Autodesk Fusion 360 part; units mm, degrees
note: some values were not read from the file. Chosen so that the rebuilt part matches the saved one: which bodies a step acts on; which face or edge a step refers to. Set by a fixed rule: which sketch regions a step uses.
(part 2 of 2)
sketch "Sketch18" plane through (0, 0, 282) normal (0, 0, 1) x (1, 0, 0)
  line L0 (0.3171, 299.31) -> (-8.3702, 323.1782)
  line L1 (-8.3702, 323.1782) -> (15.4979, 331.8655)
  line L2 (15.4979, 331.8655) -> (24.1853, 307.9973)
  line L3 (23.3949, 293.8753) -> (29.573, 307.8136)
  line L4 (29.573, 307.8136) -> (18.4863, 338.2741)
  line L5 (18.4863, 338.2741) -> (-14.7788, 326.1666)
  line L6 (-14.7788, 326.1666) -> (-3.6921, 295.7061)
  line L7 (-3.6921, 295.7061) -> (10, 289)
  line L8 (19.5766, 262.6886) -> (13.3984, 248.7503)
  line L9 (13.3984, 248.7503) -> (24.4851, 218.2899)
  line L10 (24.4851, 218.2899) -> (57.7502, 230.3974)
  line L11 (57.7502, 230.3974) -> (46.6635, 260.8578)
  line L12 (46.6635, 260.8578) -> (32.9714, 267.5639)
  line L13 (42.6543, 257.2539) -> (51.3417, 233.3857)
  line L14 (51.3417, 233.3857) -> (27.4735, 224.6984)
  line L15 (27.4735, 224.6984) -> (18.7862, 248.5666)
  line L16 (22.4806, 294.2806) -> (28.4955, 307.8504)
  line L17 (28.4955, 307.8504) -> (17.8886, 336.9924)
  line L18 (17.8886, 336.9924) -> (-13.4971, 325.5689)
  line L19 (-13.4971, 325.5689) -> (-2.8903, 296.4269)
  line L20 (-2.8903, 296.4269) -> (10.4399, 289.8981)
  line L21 (21.5664, 294.6858) -> (27.4179, 307.8871)
  line L22 (27.4179, 307.8871) -> (17.291, 335.7107)
  line L23 (17.291, 335.7107) -> (-12.2154, 324.9712)
  line L24 (-12.2154, 324.9712) -> (-2.0884, 297.1477)
  line L25 (-2.0884, 297.1477) -> (10.8797, 290.7961)
  line L26 (20.6522, 295.091) -> (26.3404, 307.9238)
  line L27 (26.3404, 307.9238) -> (16.6933, 334.4289)
  line L28 (16.6933, 334.4289) -> (-10.9337, 324.3735)
  line L29 (-10.9337, 324.3735) -> (-1.2866, 297.8685)
  line L30 (-1.2866, 297.8685) -> (11.3196, 291.6942)
  line L31 (19.738, 295.4962) -> (25.2628, 307.9606)
  line L32 (25.2628, 307.9606) -> (16.0956, 333.1472)
  line L33 (16.0956, 333.1472) -> (-9.652, 323.7759)
  line L34 (-9.652, 323.7759) -> (-0.4848, 298.5892)
  line L35 (-0.4848, 298.5892) -> (11.7594, 292.5923)
  line L36 (19.738, 295.4962) -> (23.3949, 293.8753)
  line L37 (11.7594, 292.5923) -> (10, 289)
  line L38 (21.0393, 262.0402) -> (15.1225, 248.6915)
  line L39 (15.1225, 248.6915) -> (25.4414, 220.3406)
  line L40 (25.4414, 220.3406) -> (55.6995, 231.3536)
  line L41 (55.6995, 231.3536) -> (45.3806, 259.7046)
  line L42 (45.3806, 259.7046) -> (32.2676, 266.127)
  line L43 (22.5021, 261.3919) -> (16.8466, 248.6327)
  line L44 (16.8466, 248.6327) -> (26.3977, 222.3913)
  line L45 (26.3977, 222.3913) -> (53.6487, 232.3099)
  line L46 (53.6487, 232.3099) -> (44.0977, 258.5513)
  line L47 (44.0977, 258.5513) -> (31.5639, 264.6901)
  line L48 (23.9648, 260.7435) -> (18.5706, 248.574)
  line L49 (18.5706, 248.574) -> (27.3539, 224.4421)
  line L50 (27.3539, 224.4421) -> (51.598, 233.2662)
  line L51 (51.598, 233.2662) -> (42.8147, 257.3981)
  line L52 (42.8147, 257.3981) -> (30.8601, 263.2532)
  line L53 (25.4275, 260.0952) -> (20.2947, 248.5152)
  line L54 (20.2947, 248.5152) -> (28.3102, 226.4928)
  line L55 (28.3102, 226.4928) -> (49.5473, 234.2225)
  line L56 (49.5473, 234.2225) -> (41.5318, 256.2448)
  line L57 (41.5318, 256.2448) -> (30.1563, 261.8163)
  line L58 (30.1563, 261.8163) -> (32.9714, 267.5639)
  line L59 (25.4275, 260.0952) -> (19.5766, 262.6886)
  line L60 (24.1853, 307.9973) -> (18.8238, 295.9015)
  line L61 (18.8238, 295.9015) -> (19.738, 295.4962)
  line L62 (0.3171, 299.31) -> (12.1993, 293.4903)
  line L63 (12.1993, 293.4903) -> (11.7594, 292.5923)
  line L64 (25.4275, 260.0952) -> (24.1476, 260.6625)
  line L65 (24.1476, 260.6625) -> (18.7862, 248.5666)
  line L66 (30.1563, 261.8163) -> (30.7721, 263.0736)
  line L67 (30.7721, 263.0736) -> (42.6543, 257.2539)
  dimension "d128" = 1
  dimension "d129" = 2
  dimension "d130" = 3
  dimension "d131" = 4
  dimension "d132" = 1.6
  dimension "d133" = 3.2
  dimension "d134" = 4.8
  dimension "d135" = 6.4
extrude "Extrude26" add sketch "Sketch18" against normal up to surface (127 mm away) separate body contours L3 L4 L5 L6 L7 L16 L17 L18 L19 L20 L36 L37 | L8 L9 L10 L11 L12 L38 L39 L40 L41 L42 L58 L59 makes body 48 at (7.3979, 334.2382, 239.6667) makes body 49 at (35.5735, 222.3257, 239.6667)
delete_body "RemoveBody32" bodies 23
delete_body "RemoveBody33" bodies 18
extrude "Extrude27" add sketch "Sketch18" against normal up to surface (127 mm away) separate body contours L16 L17 L18 L19 L20 L21 L22 L23 L24 L25 L36 L37 | L38 L39 L40 L41 L42 L43 L44 L45 L46 L47 L58 L59 makes body 50 at (35.5274, 224.0116, 239.6667) makes body 51 at (7.4267, 333.1845, 239.6667)
extrude "Extrude28" add sketch "Sketch18" against normal up to surface (127 mm away) separate body contours L21 L22 L23 L24 L25 L26 L27 L28 L29 L30 L36 L37 | L43 L44 L45 L46 L47 L48 L49 L50 L51 L52 L58 L59 makes body 52 at (7.4555, 332.1308, 197.3333) makes body 53 at (35.4814, 225.6975, 239.6667)
extrude "Extrude29" add sketch "Sketch18" against normal up to surface (127 mm away) separate body contours L26 L27 L28 L29 L30 L31 L32 L33 L34 L35 L36 L37 | L13 L14 L15 L48 L49 L50 L51 L52 L58 L59 L65 L67 | L13 L14 L15 L53 L54 L55 L56 L57 L58 L59 L64 L65 L66 L67 makes body 54 at (35.4353, 227.3834, 239.6667) makes body 55 at (7.4843, 331.0771, 239.6667)
extrude "Extrude30" add sketch "Sketch18" against normal up to surface (127 mm away) separate body contours L0 L1 L2 L31 L32 L33 L34 L35 L60 L61 L62 L63 | L13 L14 L15 L53 L54 L55 L56 L57 L58 L59 L64 L65 L66 L67 makes body 56 at (43.3856, 230.49, 197.3333) makes body 57 at (7.5131, 330.0234, 239.6667)
pattern_circular "C-Pattern2" count 5 over 360 about axis through (0, 205, 400) along (0, 0, -1) of bodies 49 50 53 54 56 38 makes body 58 at (60.6403, 201.5558, 239.6667) makes body 59 at (15.4633, 146.2634, 239.6667) makes body 60 at (-61.092, 175.0129, 239.6667) makes body 61 at (-47.0346, 243.4298, 239.6667) makes body 62 at (27.4705, 176.5215, 239.6667) makes body 63 at (-18.5958, 170.0737, 239.6667) makes body 64 at (-38.9633, 211.8928, 239.6667) makes body 65 at (-5.4849, 244.1863, 239.6667) makes body 66 at (65.9944, 193.5013, 197.3333) makes body 67 at (9.3658, 139.2077, 239.6667) makes body 68 at (-51.8857, 173.5273, 239.6667) makes body 69 at (-46.2488, 252.7221, 239.6667) makes body 70 at (64.1194, 189.3133, 239.6667) makes body 71 at (4.8951, 139.1714, 239.6667) makes body 72 at (-61.094, 180.0024, 239.6667) makes body 73 at (-42.6533, 255.3792, 197.3333) makes body 74 at (32.238, 178.2159, 239.6667) makes body 75 at (-15.5111, 166.0631, 239.6667) makes body 76 at (-41.8244, 207.7198, 197.3333) makes body 77 at (-10.3378, 245.6178, 239.6667) makes body 78 at (52.4522, 193.9243, 239.6667) makes body 79 at (5.675, 151.6925, 239.6667) makes body 80 at (-48.9448, 183.1298, 239.6667) makes body 81 at (-35.9245, 244.791, 197.3333)
pattern_circular "C-Pattern3" count 12 over 360 about axis through (0, 205, 400) along (0, 0, -1) of bodies 57 55 52 51 48 32 makes body 82 at (71.0259, 313.2246, 239.6667) makes body 83 at (115.6226, 263.2123, 239.6667) makes body 84 at (129.2382, 197.6021, 239.6667) makes body 85 at (108.2246, 133.9741, 239.6667) makes body 86 at (58.2123, 89.3774, 239.6667) makes body 87 at (-7.3979, 75.7618, 239.6667) makes body 88 at (-71.0259, 96.7754, 239.6667) makes body 89 at (-115.6226, 146.7877, 239.6667) makes body 90 at (-129.2382, 212.3979, 239.6667) makes body 91 at (-108.2246, 276.0259, 239.6667) makes body 92 at (-58.2123, 320.6226, 239.6667) makes body 93 at (52.0435, 273.6758, 239.6667) makes body 94 at (88.4888, 230.8344, 239.6667) makes body 95 at (85.4968, 194.2669, 239.6667) makes body 96 at (68.6758, 152.9565, 197.3333) makes body 97 at (25.8344, 116.5112, 239.6667) makes body 98 at (-10.7331, 119.5032, 239.6667) makes body 99 at (-51.7669, 136.5101, 197.3333) makes body 100 at (-79.4089, 171.5467, 239.6667) makes body 101 at (-85.4968, 215.7331, 239.6667) makes body 102 at (-68.6758, 257.0435, 239.6667) makes body 103 at (-25.8344, 293.4888, 239.6667) makes body 104 at (63.1272, 272.4257, 239.6667) makes body 105 at (88.418, 231.4973, 197.3333) makes body 106 at (89.8209, 183.7383, 197.3333) makes body 107 at (67.4257, 141.8728, 197.3333) makes body 108 at (26.8287, 116.6174, 239.6667) makes body 109 at (-20.9569, 115.0441, 239.6667) makes body 110 at (-63.1272, 137.5743, 239.6667) makes body 111 at (-88.418, 178.5027, 197.3333) makes body 112 at (-89.8209, 226.2617, 197.3333) makes body 113 at (-67.4257, 268.1272, 239.6667) makes body 114 at (-33.5214, 285.4066, 239.6667) makes body 115 at (53.7034, 274.7915, 239.6667) makes body 116 at (81.4043, 238.5895, 239.6667) makes body 117 at (87.2929, 193.3872, 239.6667) makes body 118 at (69.7915, 151.2966, 197.3333) makes body 119 at (33.5895, 123.5957, 239.6667) makes body 120 at (-11.6128, 117.7071, 239.6667) makes body 121 at (-53.7034, 135.2085, 239.6667) makes body 122 at (-81.4043, 171.4105, 239.6667) makes body 123 at (-87.2929, 216.6128, 239.6667) makes body 124 at (-68.2337, 267.5381, 239.6667) makes body 125 at (-33.5895, 286.4043, 239.6667) makes body 126 at (68.88, 279.5075, 197.3333) makes body 127 at (96.9056, 235.0854, 197.3333) makes body 128 at (98.9654, 182.6019, 239.6667) makes body 129 at (74.5075, 136.12, 197.3333) makes body 130 at (30.0854, 108.0944, 197.3333) makes body 131 at (-22.3981, 106.0346, 197.3333) makes body 132 at (-68.88, 130.4925, 239.6667) makes body 133 at (-96.9056, 174.9146, 197.3333) makes body 134 at (-98.9654, 227.3981, 197.3333) makes body 135 at (-74.5075, 273.88, 239.6667) makes body 136 at (-30.0854, 301.9056, 239.6667) makes body 137 at (55.7676, 285.0461, 239.6667) makes body 138 at (88.3192, 246.4381, 239.6667) makes body 139 at (97.2058, 196.7269, 197.3333) makes body 140 at (80.0461, 149.2324, 197.3333) makes body 141 at (41.4381, 116.6808, 239.6667) makes body 142 at (-8.2731, 107.7942, 239.6667) makes body 143 at (-55.7676, 124.9539, 197.3333) makes body 144 at (-88.3192, 163.5619, 239.6667) makes body 145 at (-100.1016, 221.2292, 197.3333) makes body 146 at (-80.0461, 260.7676, 197.3333) makes body 147 at (-41.4381, 293.3192, 197.3333)
sketch "Sketch19" plane through (172, 0, 0) normal (1, 0, 0) x (0, 0, -1)
  line L0 (-282, 377) -> (-282, 33)
  line L1 (-282, 33) -> (-155, 33)
  line L2 (-155, 33) -> (-155, 377)
  line L3 (-155, 377) -> (-282, 377)
  line L4 (-228.5, 63) -> (-208.5, 63)
  line L5 (-208.5, 63) -> (-208.5, 83)
  line L6 (-208.5, 83) -> (-228.5, 83)
  line L7 (-228.5, 83) -> (-228.5, 63)
  line L8 (-218.5, 63) -> (-218.5, 33)
  dimension "d150" = 20
  dimension "d151" = 20
  dimension "d154" = 30
  measures "d150" distance of L4.end L5.end
  measures "d151" distance of L5.end L6.end
  measures "d154" distance of L8.start L8.end
extrude "Extrude31" add sketch "Sketch19" along normal blind 40 contours L4 L5 L6 L7 bodies 9
sketch "Sketch20" plane through (175, 0, 0) normal (1, 0, 0) x (0, 0, -1)
  line L0 (-2.5, 67) -> (-7.5, 67)
  arc A0 (-7.5, 67) -> (-7.5, 37) centre (-7.5, 52) ccw
  line L1 (-7.5, 37) -> (-2.5, 37)
  arc A1 (-2.5, 37) -> (-2.5, 67) centre (-2.5, 52) ccw
  line L2 (-2.5, 52) -> (-7.5, 52) construction
  line L3 (-5, 52) -> (-5, 30)
  arc A2 (-2.5, 38) -> (-2.5, 66) centre (-2.5, 52) ccw
  line L4 (-2.5, 66) -> (-7.5, 66)
  arc A3 (-7.5, 66) -> (-7.5, 38) centre (-7.5, 52) ccw
  line L5 (-7.5, 38) -> (-2.5, 38)
  line L6 (4.5, 49.5) -> (4.5, 54.5)
  arc A4 (4.5, 54.5) -> (1.5, 54.5) centre (3, 54.5) ccw
  line L7 (1.5, 54.5) -> (1.5, 49.5)
  arc A5 (1.5, 49.5) -> (4.5, 49.5) centre (3, 49.5) ccw
  line L8 (3, 49.5) -> (3, 54.5) construction
  line L9 (3, 52) -> (-2.5, 52)
  arc A6 (-11.5, 54.5) -> (-14.5, 54.5) centre (-13, 54.5) ccw
  line L10 (-11.5, 54.5) -> (-11.5, 49.5)
  arc A7 (-14.5, 49.5) -> (-11.5, 49.5) centre (-13, 49.5) ccw
  line L11 (-14.5, 49.5) -> (-14.5, 54.5)
  line L12 (70, 70) -> (400.4623, 70)
  arc A8 (-2.5, 73) -> (-2.5, 103) centre (-2.5, 88) ccw
  line L13 (-2.5, 73) -> (-7.5, 73)
  line L14 (-2.5, 88) -> (-7.5, 88) construction
  line L15 (-7.5, 103) -> (-2.5, 103)
  line L16 (-2.5, 74) -> (-7.5, 74)
  line L17 (3, 88) -> (-2.5, 88)
  line L18 (3, 90.5) -> (3, 85.5) construction
  line L19 (1.5, 85.5) -> (1.5, 90.5)
  line L20 (-7.5, 102) -> (-2.5, 102)
  line L21 (4.5, 90.5) -> (4.5, 85.5)
  arc A9 (-7.5, 102) -> (-7.5, 74) centre (-7.5, 88) ccw
  arc A10 (1.5, 85.5) -> (4.5, 85.5) centre (3, 85.5) ccw
  line L22 (-14.5, 90.5) -> (-14.5, 85.5)
  arc A11 (4.5, 90.5) -> (1.5, 90.5) centre (3, 90.5) ccw
  arc A12 (-7.5, 103) -> (-7.5, 73) centre (-7.5, 88) ccw
  arc A13 (-14.5, 85.5) -> (-11.5, 85.5) centre (-13, 85.5) ccw
  line L23 (-11.5, 85.5) -> (-11.5, 90.5)
  arc A14 (-11.5, 90.5) -> (-14.5, 90.5) centre (-13, 90.5) ccw
  arc A15 (-2.5, 74) -> (-2.5, 102) centre (-2.5, 88) ccw
  line L24 (-30, 30) -> (70, 30)
  line L25 (70, 30) -> (70, 110)
  line L26 (70, 110) -> (-30, 110)
  line L27 (-30, 110) -> (-30, 30)
  line L28 (-30, 30) -> (20, 30)
  point P0 (-5, 88)
  dimension "d155" = 15
  dimension "d157" = 5
  dimension "d158" = 1
  dimension "d159" = 5
  dimension "d160" = 3
  dimension "d161" = 8
  dimension "d176" = 22
  measures "d155" radius of A0
  measures "d157" distance of A1.centre A0.centre
  measures "d159" distance of A5.centre A4.centre
  measures "d160" distance of L6.start L7.end
  measures "d161" distance of L3 L8
  measures "d176" distance of L3.start L3.end
extrude "Extrude32" cut sketch "Sketch20" against normal blind 1 contours L0 A0 L1 A1 | A8 L13 L15 A12 bodies 8
extrude "Extrude33" cut sketch "Sketch20" against normal blind 10 contours L6 A4 L7 A5 | A6 L10 A7 L11 | L19 L21 A10 A11 | L22 A13 L23 A14 bodies 8
ref_plane "WorkPlane3" through (145, 70, -40) normal (0, 0, -1) x (-1, 0, 0)
sketch "Sketch21" plane through (170, 70, -40) normal (0, 0, -1) x (1, 0, 0)
  line L0 (5, 40) -> (5, -40)
  line L1 (5, -20) -> (15, -20)
  line L2 (5, 20) -> (11, 20)
  arc A0 (11, 20) -> (15, -20) centre (79.7195, 6.6719) ccw
  dimension "d168" = 6
  dimension "d169" = 10
  dimension "d170" = 20
  dimension "d171" = 20
  dimension "d172" = 70
  measures "d168" distance of L2.start L2.end
  measures "d169" distance of L1.start L1.end
  measures "d170" distance of L0.end L1
  measures "d171" distance of L0.start L2
  measures "d172" radius of A0
extrude "Extrude34" [suppressed]
sketch "Sketch22" plane through (0, 33, 0) normal (0, 1, 0) x (-1, 0, 0)
  circle A0 centre (-119.4306, -115) radius 5
  circle A1 centre (-119.4306, -385) radius 5
  line L0 (-134.4306, -397) -> (-66.2345, -397)
  line L1 (-66.2345, -397) -> (-66.2345, -103)
  line L2 (-66.2345, -103) -> (-134.4306, -103)
  line L3 (-134.4306, -103) -> (-134.4306, -397)
  line L4 (-124.3381, -123.5) -> (-114.5231, -123.5)
  line L5 (-114.5231, -123.5) -> (-109.6156, -115)
  line L6 (-109.6156, -115) -> (-114.5231, -106.5)
  line L7 (-114.5231, -106.5) -> (-124.3381, -106.5)
  line L8 (-124.3381, -106.5) -> (-129.2456, -115)
  line L9 (-129.2456, -115) -> (-124.3381, -123.5)
  point P0 (-119.4306, -115)
  dimension "d177" = 17
  measures "d177" distance of L4 L7
extrude "Extrude35" add sketch "Sketch22" along normal blind 8 separate body contours A0 | L4 L5 L6 L7 L8 L9 makes body 148
sketch "Sketch23" plane through (0, 33, 0) normal (0, -1, 0) x (1, 0, 0)
  line L0 (124.3381, -123.5) -> (129.2456, -115)
  line L1 (129.2456, -115) -> (124.3381, -106.5)
  line L2 (124.3381, -106.5) -> (114.5231, -106.5)
  line L3 (114.5231, -106.5) -> (109.6156, -115)
  line L4 (109.6156, -115) -> (114.5231, -123.5)
  line L5 (114.5231, -123.5) -> (124.3381, -123.5)
  circle A0 centre (119.4306, -115) radius 5
extrude "Extrude36" add sketch "Sketch23" along normal blind 45 contours A0 bodies 148
sketch "Sketch24" plane through (0, 0, 0) normal (0, -1, 0) x (1, 0, 0)
  circle A0 centre (119.4306, -115) radius 5
  circle A1 centre (119.4306, -385) radius 5
  circle A2 centre (-120, -115) radius 5
  circle A3 centre (-120, -385) radius 5
  line L0 (145, -370) -> (175, -370)
  line L1 (175, -370) -> (175, 370)
  line L2 (175, 370) -> (145, 370)
  line L3 (145, 370) -> (145, -100)
  line L4 (145, -100) -> (25, -100)
  line L5 (25, -100) -> (25, 370)
  line L6 (25, 370) -> (145, 370)
  line L7 (145, 370) -> (145, 400)
  line L8 (145, 400) -> (-145, 400)
  line L9 (-145, 400) -> (-145, 370)
  line L10 (-145, 370) -> (-25, 370)
  line L11 (-25, 370) -> (-25, -100)
  line L12 (-25, -100) -> (-145, -100)
  line L13 (-145, -100) -> (-145, 370)
  line L14 (-145, 370) -> (-175, 370)
  line L15 (-175, 370) -> (-175, -370)
  line L16 (-175, -370) -> (-145, -370)
  line L17 (-145, -370) -> (-145, -130)
  line L18 (-145, -130) -> (-25, -130)
  line L19 (-25, -130) -> (-25, -370)
  line L20 (-25, -370) -> (-145, -370)
  line L21 (-145, -370) -> (-145, -400)
  line L22 (-145, -400) -> (145, -400)
  line L23 (145, -400) -> (145, -370)
  line L24 (145, -370) -> (25, -370)
  line L25 (25, -370) -> (25, -130)
  line L26 (25, -130) -> (145, -130)
  line L27 (145, -130) -> (145, -370)
  line L28 (129.2456, -115) -> (124.3381, -123.5)
  line L29 (124.3381, -123.5) -> (114.5231, -123.5)
  line L30 (114.5231, -123.5) -> (109.6156, -115)
  line L31 (109.6156, -115) -> (114.5231, -106.5)
  line L32 (114.5231, -106.5) -> (124.3381, -106.5)
  line L33 (124.3381, -106.5) -> (129.2456, -115)
extrude "Extrude37" add sketch "Sketch24" along normal blind 8 separate body contours L28 L29 L30 L31 L32 L33 makes body 149
ref_plane "WorkPlane4" through (0, 205, -250) normal (0, 0, -1) x (-1, 0, 0)
mirror "Mirror2" about plane through (0, 205, -250) normal (0, 0, -1) of bodies 148 149 makes body 150 at (119.5552, 0, -377.6713) makes body 151 at (124.3315, 3, -384.0093)
mirror "Mirror3" about plane through (0, 0, 0) normal (1, 0, 0) of bodies 149 148 150 151 makes body 152 at (-119.5552, 0, -122.3287) makes body 153 at (-124.3315, 3, -384.0093) makes body 154 at (-119.5552, 0, -377.6713) makes body 155 at (-124.4244, 3, -115.2492)
delete_body "RemoveBody34" bodies 6
sketch "Sketch25" plane through (0, 110, 0) normal (0, 1, 0) x (-1, 0, 0)
  line L0 (-175, -70) -> (-115, -70)
  line L1 (-115, -70) -> (-115, 30)
  line L2 (-115, 30) -> (-175, 30)
  line L3 (-175, 30) -> (-175, -70)
  circle A0 centre (-145, -45) radius 7.5
  point P0 (-145, -70)
  dimension "d186" = 15
  dimension "d187" = 25
  measures "d186" diameter of A0
  measures "d187" distance of A0.centre P0
extrude "Extrude38" add sketch "Sketch25" along normal blind 15 contours A0 bodies 8
sketch "Sketch26" plane through (0, 0, 0) normal (1, 0, 0) x (0, 0, -1)
  circle A0 centre (133, 223.647) radius 7.5
  point P0 (103, 223.647)
  dimension "d190" = 15
  dimension "d191" = 30
  measures "d190" diameter of A0
  measures "d191" distance of A0.centre P0
extrude "Extrude39" add sketch "Sketch26" along normal blind 115 bodies 5
sketch "Sketch27" plane through (0, 0, 0) normal (1, 0, 0) x (0, 0, -1)
  circle A0 centre (133, 223.647) radius 7.5
  line L0 (52.5, 125) -> (37.5, 125)
  spline S0 degree 5 poles (45, 125) (45, 129.2029) (46.1969, 137.7196) (51.5794, 150.8264) (64.8013, 168.7214) (87.0471, 190.4721) (106.1967, 205.9765) (119.9809, 215.6951) (128.7333, 221.1647) (133, 223.647) knots 0 0 0 0 0 0 0.2 0.4 0.6 0.8 1 1 1 1 1 1
  line L1 (45, 115.4893) -> (45, 134.5107)
  line L2 (122.3818, 217.4697) -> (143.6182, 229.8242)
  point P0 (45, 125)
sketch "Sketch28" plane through (0, 0, 0) normal (0, 0, 1) x (1, 0, 0)
  line L0 (115, 216.147) -> (115, 231.147)
  line L1 (152.5, 125) -> (137.5, 125)
  spline S0 degree 5 poles (145, 125) (145, 127.4293) (144.95, 133.4038) (144.7246, 145.7096) (143.9179, 167.3283) (140.598, 196.2083) (134.2343, 214.452) (126.1328, 221.9742) (118.9999, 223.647) (115, 223.647) knots 0 0 0 0 0 0 0.2 0.4 0.6 0.8 1 1 1 1 1 1
  line L2 (145, 118.9364) -> (145, 131.0636)
  line L3 (122.5301, 223.647) -> (107.4699, 223.647)
  point P0 (115, 223.647)
sketch "Sketch29" plane through (0, 0, 0) normal (0, 0, 1) x (1, 0, 0)
  spline S0 degree 3 poles (115, 223.647, -133) (116.5147, 223.647, -133) (117.9658, 223.5036, -132.7523) (120.8091, 222.9007, -131.7268) (122.1051, 222.4486, -130.9638) (125.0601, 221.0644, -128.6782) (126.5666, 219.9873, -126.944) (130.0874, 216.832, -122.0357) (132.1388, 214.1005, -117.9573) (137.7605, 203.205, -102.9477) (140.1148, 193.322, -90.7451) (142.8972, 174.107, -70.8414) (143.7281, 164.2794, -61.8111) (144.5044, 148.9467, -51.8351) (144.7089, 143.2422, -48.818) (144.9328, 133.2913, -45.7171) (145, 129.1933, -45) (145, 125, -45) knots 0 0 0 0 0.45439509 0.45439509 0.92496171 0.92496171 1.65100835 1.65100835 2.97408854 2.97408854 5.70884665 5.70884665 7.82525926 7.82525926 8.90996943 8.90996943 9.64044951 9.64044951 9.64044951 9.64044951
  point P0 (145, 125)
pipe "Pipe1" add diameter 10 path "Sketch29" along S0 separate body makes body 156
combine "Combine2" operation add target body 44 tool bodies 4
combine "Combine3" operation add target body 1 tool bodies 2 3
equation "d37 = d38"
equation "d66 = d65"
equation "d71 = d70"
equation "d72 = d70"
equation "d73 = d71"
equation "d151 = d150"
equation "d171 = d170"
named bodies: "transparent", "holder", "metal", "holder i"
